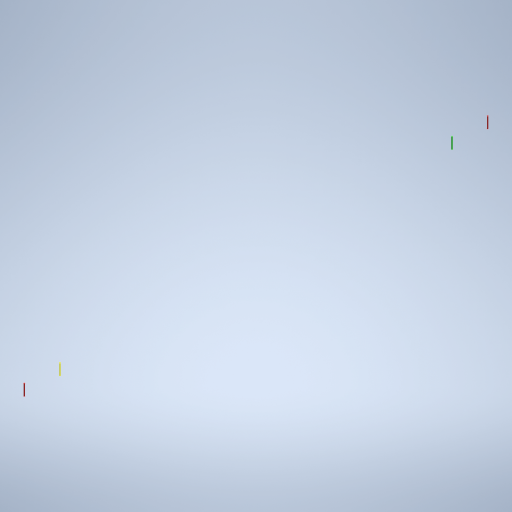
# Autodesk Inventor part: Minifix&Dowel Joint 11200
Saved by Autodesk Inventor 2024 (Build 280153000, 153)
## iProperties
RuleStatus: InUse
Created: 2023-01-09
Part Number: Minifix&Dowel Joint 11200
Material: Generic
Document SubType Name: Modeling
Designer: sauliusd
Density: 1 g/cm^3
Appearance: Default
AfterAnyUserParamChange0: ComponenetsArrayParams
AfterAnyParamChange0: ComponenetsArrayParams
Author: sauliusd
Autodesk Inventor part; units mm, degrees
ref_plane "YZ Plane" through (0, 0, 0) normal (1, 0, 0) x (0, 1, 0)
ref_plane "XZ Plane" through (0, 0, 0) normal (0, 1, 0) x (-1, 0, 0)
ref_plane "XY Plane" through (0, 0, 0) normal (0, 0, 1) x (1, 0, 0)
sketch "Sketch1" plane through (0, 0, 0) normal (0, 0, 1) x (1, 0, 0)
  line L0 (-300, -9) -> (300, -9)
  line L1 (300, -9) -> (300, 9)
  line L2 (300, 9) -> (-300, 9)
  line L3 (-300, 9) -> (-300, -9)
  line L4 (-300, -9) -> (300, 9) construction
  line L5 (300, -9) -> (-300, 9) construction
  point P0 (0, 0)
  dimension "d0" = 600
  dimension "d1" = 18
  constraints: 12 end point, 2 midpoint, 2 parallel, 1 horizontal, 1 perpendicular
  measures "d0" distance of L2.end L1.end
  measures "d1" distance of L0.end L1.end
sketch "Sketch2" plane through (0, 0, 0) normal (0, 0, 1) x (1, 0, 0)
  circle A0 centre (238, -0.5) radius 0.5
  line L0 (300, 9) -> (-300, 9) projected
  line L1 (-300, -9) -> (300, -9) projected
  line L2 (0, -12.6) -> (0, 12.6) projected
  line L3 (300, -9) -> (300, 9) projected
  point P0 (0, 0)
  dimension "d3" = 9.5
  dimension "d4" = 1
  dimension "d26" = 62
  constraints: 1 centre point
  measures "d3" distance from line of L0 A0.centre
  measures "d4" diameter of A0
  measures "d26" distance from line of L3 A0.centre
extrude "Extrusion1" add sketch "Sketch2" along normal blind 10 contours A0
pattern_linear "Minifix Array" count 2 spacing 416 along (-1, 0, 0) of "Extrusion1"
sketch "Sketch3" plane through (0, 0, 0) normal (0, 0, 1) x (1, 0, 0)
  circle A0 centre (206, -0.5) radius 0.5
  circle A1 centre (238, -0.5) radius 0.5 projected
  point P0 (0, 0)
  dimension "d11" = 32
  constraints: 1 centre point, 1 equal radius, 1 horizontal alignment
  measures "d11" distance of A1.centre A0.centre
extrude "Extrusion2" add sketch "Sketch3" along normal blind 10 separate body contours A0
pattern_of_one "Left Dowel Array" bodies 2
sketch "Sketch4" plane through (0, 0, 0) normal (0, 0, 1) x (1, 0, 0)
  line L0 (-300, 9) -> (-300, -9) projected
  circle A0 centre (-146, -0.5) radius 0.5
  circle A1 centre (238, -0.5) radius 0.5 projected
  line L1 (300, -9) -> (300, 9) projected
  point P0 (0, 0)
  dimension "d17" = 62
  dimension "d28" = 446
  constraints: 1 centre point, 1 equal radius, 1 horizontal alignment
  measures "d17" distance from line of L1 A1.centre
  measures "d28" distance from line of L1 A0.centre
extrude "Extrusion3" add sketch "Sketch4" along normal blind 10 separate body contours A0
pattern_of_one "Right Dowel Array" bodies 3
equation "\"d3\" = Y_Coord"
equation "\"d26\" = X_Coord"
equation "\"d9\" = Step"
equation "\"d16\" = Step"
equation "\"d28\" = PlacingWithByStep + X_Coord - PlacingStep"
equation "\"d23\" = Step"
equation "\"d0\" = ContactPatchWidth"
equation "\"d1\" = ContactPatchHeight"
equation "\"ContactPatchWidth\" = 600"
equation "\"ContactPatchHeight\" = 18"
equation "\"PlacingStep\" = 32"
equation "\"PlacingWithByStep\" = 416"
equation "\"X_Coord\" = 62"
equation "\"Step\" = 416"
equation "\"Y_Coord\" = 9.5"
equation "\"MaxDistBetweenByStep\" = 192"
